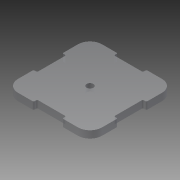
# Autodesk Inventor part: 290814 Forward Outer Endcap
Saved by Autodesk Inventor 2015 (Build 190159000, 159)
## iProperties
Created: 2013-05-23
Part Number: 290814 Forward Outer Endcap
Material: Polycarbonate, Clear
Document SubType Name: Modeling
Designer: Eric
Density: 1.2 g/cm^3
Mass: 2.90508 g
Surface Area: 20.2664 cm^2
Volume: 2.4209 cm^3
Appearance: Polycarbonate - Clear
Author: Eric
Autodesk Inventor part; units mm, degrees
ref_plane "YZ Plane" through (0, 0, 0) normal (1, 0, 0) x (0, 1, 0)
ref_plane "XZ Plane" through (0, 0, 0) normal (0, 1, 0) x (-1, 0, 0)
ref_plane "XY Plane" through (0, 0, 0) normal (0, 0, 1) x (1, 0, 0)
sketch "Sketch1" plane through (0, 0, 0) normal (0, 0, 1) x (1, 0, 0)
  circle A0 centre (0, 0) radius 16 construction
  line L0 (17.5, 17.5) -> (-17.5, -17.5) construction
  line L1 (-17.5, 17.5) -> (17.5, -17.5) construction
  line L2 (-17, -6) -> (-16.5, -6)
  line L3 (-16, -5.5) -> (-16, 5.5)
  line L4 (-16.5, 6) -> (-17, 6)
  line L5 (-17.5, 12.5) -> (-17.5, 6.5)
  line L6 (-17.5, -6.5) -> (-17.5, -12.5)
  arc A1 (-16.5, -6) -> (-16, -5.5) centre (-16.5, -5.5) ccw
  arc A2 (-16, 5.5) -> (-16.5, 6) centre (-16.5, 5.5) ccw
  arc A3 (-17.5, 6.5) -> (-17, 6) centre (-17, 6.5) ccw
  arc A4 (-17, -6) -> (-17.5, -6.5) centre (-17, -6.5) ccw
  line L7 (6, -17) -> (6, -16.5)
  line L8 (5.5, -16) -> (-5.5, -16)
  line L9 (-6, -16.5) -> (-6, -17)
  arc A5 (6, -16.5) -> (5.5, -16) centre (5.5, -16.5) ccw
  arc A6 (-5.5, -16) -> (-6, -16.5) centre (-5.5, -16.5) ccw
  arc A7 (-6.5, -17.5) -> (-6, -17) centre (-6.5, -17) ccw
  arc A8 (6, -17) -> (6.5, -17.5) centre (6.5, -17) ccw
  line L10 (17, 6) -> (16.5, 6)
  line L11 (16, 5.5) -> (16, -5.5)
  line L12 (16.5, -6) -> (17, -6)
  arc A9 (16.5, 6) -> (16, 5.5) centre (16.5, 5.5) ccw
  arc A10 (16, -5.5) -> (16.5, -6) centre (16.5, -5.5) ccw
  arc A11 (17.5, -6.5) -> (17, -6) centre (17, -6.5) ccw
  arc A12 (17, 6) -> (17.5, 6.5) centre (17, 6.5) ccw
  line L13 (-6, 17) -> (-6, 16.5)
  line L14 (-5.5, 16) -> (5.5, 16)
  line L15 (6, 16.5) -> (6, 17)
  arc A13 (-6, 16.5) -> (-5.5, 16) centre (-5.5, 16.5) ccw
  arc A14 (5.5, 16) -> (6, 16.5) centre (5.5, 16.5) ccw
  arc A15 (6.5, 17.5) -> (6, 17) centre (6.5, 17) ccw
  arc A16 (-6, 17) -> (-6.5, 17.5) centre (-6.5, 17) ccw
  line L16 (12.5, 17.5) -> (6.5, 17.5)
  line L17 (-6.5, 17.5) -> (-12.5, 17.5)
  line L18 (17.5, -12.5) -> (17.5, -6.5)
  line L19 (17.5, 6.5) -> (17.5, 12.5)
  line L20 (-12.5, -17.5) -> (-6.5, -17.5)
  line L21 (6.5, -17.5) -> (12.5, -17.5)
  arc A17 (-17.5, -12.5) -> (-12.5, -17.5) centre (-12.5, -12.5) ccw
  arc A18 (-12.5, 17.5) -> (-17.5, 12.5) centre (-12.5, 12.5) ccw
  arc A19 (17.5, 12.5) -> (12.5, 17.5) centre (12.5, 12.5) ccw
  arc A20 (12.5, -17.5) -> (17.5, -12.5) centre (12.5, -12.5) ccw
  circle A21 centre (0, 0) radius 1.4
  point P0 (16, 0)
  point P1 (0, 0)
  point P2 (-16, 6)
  point P3 (-16, -6)
  point P4 (-16, 0)
  point P5 (-6, -16)
  point P6 (6, -16)
  point P7 (0, -16)
  point P8 (16, -6)
  point P9 (16, 6)
  point P10 (6, 16)
  point P11 (-6, 16)
  point P12 (0, 16)
  dimension "d17" = 16
  dimension "d39" = 35
  dimension "d44" = 12
  dimension "d45" = 0.5
  dimension "d48" = 360
  dimension "d50" = 5
  dimension "d53" = 2.8
  constraints: 44 end point, 42 point on circle, 24 point on line, 22 centre point, 17 tangent, 9 parallel, 6 equal radius, 5 midpoint, 5 perpendicular, 4 coincident, 3 horizontal, 1 horizontal alignment, 89 other
  measures "d17" radius of A0
  measures "d39" distance of L1.end L0.start
  measures "d44" distance of point (-16, -6) point (-16, 6)
  measures "d45" radius of A1
  measures "d50" radius of A17
  measures "d53" diameter of A21
extrude "Extrusion6" add sketch "Sketch1" along normal blind 3
body "Solid6"
